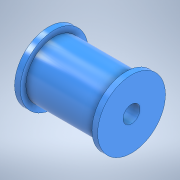
# Autodesk Inventor part: HubV2
Saved by Autodesk Inventor 2020 (Build 240168000, 168)
## iProperties
Created: 2023-11-28
Part Number: HubV2
Material: Generic
Document SubType Name: Modeling
Designer: smz3rm
Mass: 5.6 g
Surface Area: 8.94097 cm^2
Volume: 1.11974 cm^3
Density: 5.00115 g/cm^3
Appearance: Cyan
Author: smz3rm
Autodesk Inventor part; units mm, degrees
ref_plane "YZ Plane" through (0, 0, 0) normal (1, 0, 0) x (0, 1, 0)
ref_plane "XZ Plane" through (0, 0, 0) normal (0, 1, 0) x (-1, 0, 0)
ref_plane "XY Plane" through (0, 0, 0) normal (0, 0, 1) x (1, 0, 0)
sketch "Sketch1" plane through (0, 0, 0) normal (1, 0, 0) x (0, 1, 0)
  circle A0 centre (0, 0) radius 1.5
  circle A1 centre (0, 0) radius 5
  dimension "d0" = 3
  dimension "d1" = 10
  constraints: 2 centre point, 2 coincident
  measures "d0" diameter of A0
  measures "d1" diameter of A1
extrude "Extrusion1" add sketch "Sketch1" along normal mid plane 12.7
sketch "Sketch2" plane through (6.35, 0, 0) normal (1, 0, 0) x (0, 0, -1)
  circle A0 centre (0, 0) radius 6
  circle A1 centre (0, 0) radius 1.5
  dimension "d4" = 12
  dimension "d5" = 3
  constraints: 2 centre point, 2 coincident
  measures "d4" diameter of A0
  measures "d5" diameter of A1
extrude "Extrusion2" add sketch "Sketch2" along normal blind 1
mirror "Mirror1" about plane through (0, 0, 0) normal (1, 0, 0) of "Extrusion2"
body "Solid1"
